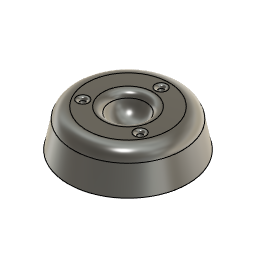
Snap Shine Final Assemply (Autodesk Fusion 360 archive; units mm, degrees)
design "Base"
description: Mounts to wall
Autodesk Fusion 360 part; units mm, degrees
note: some values were not read from the file. Chosen so that the rebuilt part matches the saved one: which bodies a step acts on; a side. Set by a fixed rule: the direction of a hole.
sketch "Sketch3" plane through (0, 0, 0) normal (0, 0, 1) x (1, 0, 0)
  circle A0 centre (0, 0) radius 40
  dimension "d10" = 80
  constraint coincident A0.centre origin
  measures "d10" diameter of A0
ref_plane "WorkPlane2" through (0, 0, 25) normal (0, 0, 1) x (1, 0, 0)
sketch "Sketch5" plane through (0, 0, 25) normal (0, 0, 1) x (1, 0, 0)
  circle A0 centre (0, 0) radius 35
  dimension "d12" = 70
  constraint coincident A0.centre origin
  measures "d12" diameter of A0
loft "Loft1" add profiles "Sketch5", "Sketch3" section 1 section 2
fillet "Fillet4" radius 9 1 edges at (-32.6315, 12.6565, 25)
ref_plane "WorkPlane3" through (0, 0, 25) normal (0, 0, 1) x (1, 0, 0)
sphere "SpherePrimitive2" cut diameter 25 placed x (1, 0, 0) y (0, 1, 0) z (0, 0, 1) at (0, 0, 25)
fillet "Fillet5" radius 5 1 edges at (-4.5202, -11.6541, 25)
sketch "Sketch8" plane through (0, 0, 25) normal (0, 0, 1) x (-1, 0, 0)
  circle A0 centre (0, 0) radius 27.6218
  circle A1 centre (0, 0) radius 16.7705
  circle A2 centre (0, -22.196) radius 1.8885
  circle A3 centre (19.2223, 11.098) radius 1.8885
  circle A4 centre (-19.2223, 11.098) radius 1.8885
  point P0 (19.2223, 11.098)
  point P1 (-19.2223, 11.098)
  dimension "d33" = 3.777
  dimension "d36" = 3.777
  dimension "d37" = 3.777
  dimension "d38" = 22.196
  dimension "d39" = 19.2223
  dimension "d40" = 11.098
  dimension "d41" = 19.2223
  dimension "d42" = 11.098
  constraint coincident P0 A3.centre
  constraint coincident P1 A4.centre
  constraint vertical A0.centre A2.centre
  measures "d33" diameter of A2
  measures "d36" diameter of A3
  measures "d37" diameter of A4
  measures "d38" distance of A0.centre A2.centre
  measures "d39" horizontal distance of A0.centre A3.centre
  measures "d40" vertical distance of A0.centre A3.centre
  measures "d41" horizontal distance of A0.centre P1
  measures "d42" vertical distance of A0.centre P1
extrude "Extrude2" cut sketch "Sketch8" against normal blind 35 contours A2 | A3 | A4
fillet "Fillet6" radius 2 3 edges at (1.7607, 21.5131, 25) (20.983, -11.7809, 25) (-17.4616, -11.7809, 25)
sketch "Sketch11" plane through (0, 0, 0) normal (0, 0, -1) x (1, 0, 0)
  circle A0 centre (0, -22.196) radius 1.8885
  circle A1 centre (19.2223, 11.098) radius 1.8885
  circle A2 centre (-19.2223, 11.098) radius 1.8885
  circle A3 centre (0, 0) radius 40
  line L0 (3.175, 10.175) -> (-3.175, 10.175)
  line L1 (-3.175, 10.175) -> (-3.175, 3.825)
  line L2 (-3.175, 3.825) -> (3.175, 3.825)
  line L3 (3.175, 3.825) -> (3.175, 10.175)
  line L4 (3.175, 10.175) -> (-3.175, 3.825) construction
  line L5 (-3.175, 10.175) -> (3.175, 3.825) construction
  line L6 (-7.2243, -7.8372) -> (-1.725, -4.6622)
  line L7 (-10.3993, -2.3379) -> (-7.2243, -7.8372)
  line L8 (-4.9, 0.8371) -> (-10.3993, -2.3379)
  line L9 (-1.725, -4.6622) -> (-4.9, 0.8371)
  line L10 (10.3993, -2.3378) -> (4.9001, 0.8372)
  line L11 (7.2243, -7.8371) -> (10.3993, -2.3378)
  line L12 (1.7251, -4.6621) -> (7.2243, -7.8371)
  line L13 (4.9001, 0.8372) -> (1.7251, -4.6621)
  point P0 (0, 7)
  point P1 (-6.0622, -3.5)
  point P2 (6.0622, -3.5)
  dimension "d50" = 6.35
  dimension "d51" = 6.35
  dimension "d52" = 7
  dimension "d54" = 360
  constraint horizontal L0
  constraint perpendicular L0 L1
  constraint parallel L0 L2
  constraint parallel L1 L3
  constraint coincident L4 P0
  constraint coincident L5 P0
  measures "d50" distance of L1.end L2.end
  measures "d51" distance of L0.end L1.end
  measures "d52" distance of A3.centre P0
extrude "Extrude4" cut sketch "Sketch11" against normal blind 6.35 contours L0 L1 L2 L3 | L6 L7 L8 L9 | L10 L11 L12 L13

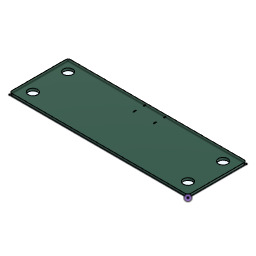
design "circuit board"
description: Cicuit Board for Lamp
Autodesk Fusion 360 part; units mm, degrees
sketch "Sketch1" plane through (0, 0, 0) normal (0, 0, 1) x (1, 0, 0)
  line L0 (0, 0) -> (-76.2, 0)
  line L1 (-76.2, 0) -> (-76.2, 25)
  line L2 (-76.2, 25) -> (0, 25)
  line L3 (0, 25) -> (0, 0)
  dimension "d1" = 76.2
  dimension "d2" = 25
  constraint horizontal L0
  constraint vertical L1
  constraint horizontal L2
  constraint vertical L3
  constraint coincident L0.start L3.end
  measures "d1" distance of L1.end L2.end
  measures "d2" distance of L0.end L1.end
extrude "Extrude1" add sketch "Sketch1" along normal blind 1
fillet "Fillet1" radius 1 4 edges at (0, 0, 0.5) (0, 25, 0.5) (-76.2, 25, 0.5) (-76.2, 0, 0.5)
sketch "Sketch2" plane through (0, 0, 1) normal (0, 0, 1) x (-1, 0, 0)
  arc A0 (76.2, -1) -> (75.2, 0) centre (75.2, -1) ccw
  line L0 (75.2, 0) -> (1, 0)
  arc A1 (1, 0) -> (0, -1) centre (1, -1) ccw
  line L1 (0, -1) -> (0, -24)
  arc A2 (0, -24) -> (1, -25) centre (1, -24) ccw
  line L2 (1, -25) -> (75.2, -25)
  arc A3 (75.2, -25) -> (76.2, -24) centre (75.2, -24) ccw
  line L3 (76.2, -24) -> (76.2, -1)
  point P0 (5, -5)
  dimension "d7" = 5
  dimension "d8" = 5
  measures "d7" horizontal distance of origin P0
  measures "d8" vertical distance of origin P0
hole "Hole1" at (-5, 5, 1) direction (0, 0, -1) diameter 4 end through all
pattern_linear "R-Pattern1" count 2 spacing 66.2 along (-1, 0, 0) count 2 spacing 15 along (0, 1, 0) of "Hole1"
sketch "Sketch5" plane through (0, 0, 0) normal (0, 0, -1) x (1, 0, 0)
  circle A0 centre (-71.2, -20) radius 2
  circle A1 centre (-5, -20) radius 2
  circle A2 centre (-71.2, -5) radius 2
  circle A3 centre (-5, -5) radius 2
  arc A4 (-75.2, 0) -> (-76.2, -1) centre (-75.2, -1) ccw
  line L0 (-76.2, -1) -> (-76.2, -24)
  arc A5 (-76.2, -24) -> (-75.2, -25) centre (-75.2, -24) ccw
  line L1 (-75.2, -25) -> (-1, -25)
  arc A6 (-1, -25) -> (0, -24) centre (-1, -24) ccw
  line L2 (0, -24) -> (0, -1)
  arc A7 (0, -1) -> (-1, 0) centre (-1, -1) ccw
  line L3 (-1, 0) -> (-75.2, 0)
  line L4 (0, -23.5) -> (-76.2, -23.5)
  line L5 (-38.1, -23.5) -> (-42.27, -23.5)
  line L6 (-38.1, -23.5) -> (-33.93, -23.5)
  line L7 (-42.27, -23.5) -> (-42.57, -23.5)
  line L8 (-42.57, -23.5) -> (-42.57, -24.3)
  line L9 (-42.57, -24.3) -> (-42.27, -24.3)
  line L10 (-42.27, -24.3) -> (-42.27, -23.5)
  line L11 (-33.93, -23.5) -> (-33.63, -23.5)
  line L12 (-33.63, -23.5) -> (-33.63, -24.3)
  line L13 (-33.63, -24.3) -> (-33.93, -24.3)
  line L14 (-33.93, -24.3) -> (-33.93, -23.5)
  line L15 (-33.93, -23.5) -> (-33.93, -20.25)
  line L16 (-33.93, -20.25) -> (-33.63, -20.25)
  line L17 (-33.63, -20.25) -> (-33.63, -19.2)
  line L18 (-33.63, -19.2) -> (-33.93, -19.2)
  line L19 (-33.93, -19.2) -> (-33.93, -20.25)
  line L20 (-42.27, -23.5) -> (-42.27, -20.25)
  line L21 (-42.27, -20.25) -> (-42.57, -20.25)
  line L22 (-42.57, -20.25) -> (-42.57, -19.2)
  line L23 (-42.57, -19.2) -> (-42.27, -19.2)
  line L24 (-42.27, -19.2) -> (-42.27, -20.25)
  dimension "d57" = 1.5
  dimension "d58" = 4.17
  dimension "d59" = 4.17
  dimension "d60" = 0.3
  dimension "d61" = 0.8
  dimension "d62" = 0.3
  dimension "d63" = 0.8
  dimension "d64" = 3.25
  dimension "d65" = 0.3
  dimension "d66" = 1.05
  dimension "d67" = 3.25
  dimension "d68" = 0.3
  dimension "d69" = 1.05
  constraint coincident L2 L4.start
  constraint coincident L0 L4.end
  constraint perpendicular L0 L4
  constraint horizontal L5
  constraint midpoint L4 L5.start
  constraint parallel L4 L6
  constraint horizontal L7
  constraint vertical L8
  constraint horizontal L9
  constraint vertical L10
  constraint horizontal L11
  constraint vertical L12
  constraint horizontal L13
  constraint vertical L14
  constraint perpendicular L6 L15
  constraint horizontal L16
  constraint vertical L17
  constraint horizontal L18
  constraint vertical L19
  constraint perpendicular L7 L20
  constraint horizontal L21
  constraint vertical L22
  constraint horizontal L23
  constraint vertical L24
  measures "d57" distance of L1 L4
  measures "d58" distance of L5.start L5.end
  measures "d59" distance of L5.start L6.end
  measures "d60" distance of L5.end L7.end
  measures "d61" distance of L5.end L9.end
  measures "d62" distance of L6.end L11.end
  measures "d63" distance of L6.end L13.end
  measures "d64" distance of L6.end L15.end
  measures "d65" distance of L15.end L16.end
  measures "d66" distance of L15.end L18.end
  measures "d67" distance of L5.end L20.end
  measures "d68" distance of L20.end L21.end
  measures "d69" distance of L20.end L23.end
extrude "Extrude4" cut sketch "Sketch5" against normal through all contours L4 L7 L8 L9 L10 | L4 L11 L12 L13 L14 | L16 L17 L18 L19 | L21 L22 L23 L24

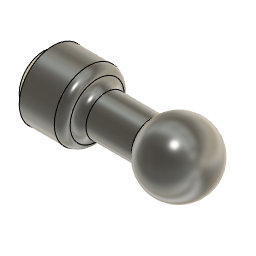
design "Ball Joint"
description: connects to base and lamp
Autodesk Fusion 360 part; units mm, degrees
sketch "Sketch1" plane through (0, 0, 0) normal (1, 0, 0) x (0, 1, 0)
  circle A0 centre (0, 0) radius 12.5
  circle A1 centre (0, 0) radius 9
  dimension "d1" = 25
  dimension "d8" = -3.5
  constraint coincident A0.centre A1.centre
  measures "d1" diameter of A0
extrude "Extrude1" add sketch "Sketch1" along normal blind 20 contours A0 | A1
sketch "Sketch2" plane through (20, 0, 0) normal (1, 0, 0) x (0, 1, 0)
  circle A0 centre (0, 0) radius 12.5
  circle A1 centre (0, 0) radius 7.5
  dimension "d4" = 15
  constraint concentric A0 A1
  measures "d4" diameter of A1
extrude "Extrude2" add sketch "Sketch2" along normal blind 30 contours A1
sphere "SpherePrimitive1" add diameter 25 placed x (0, 1, 0) y (0, 0, 1) z (1, 0, 0) at (50, 0, 0)
extrude "Extrude3" cut sketch "Sketch1" along normal blind 16.5 contours A1
chamfer "Chamfer1" distance 3.5 angle 45 1 edges at (0, -11.6541, -4.5202)
fillet "Fillet1" radius 3.5 1 edges at (20, -11.6541, -4.5202)
fillet "Fillet2" radius 3.5 1 edges at (20, -6.9925, 2.7121)

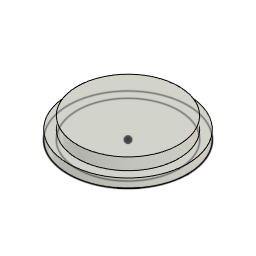
design "LED"
description: light source
Autodesk Fusion 360 part; units mm, degrees
sketch "Sketch1" plane through (0, 0, 0) normal (0, 0, 1) x (1, 0, 0)
  circle A0 centre (0, 0) radius 10
  circle A1 centre (0, 0) radius 8.5
  dimension "d1" = 20
  dimension "d2" = -1.5
  constraint coincident A0.centre A1.centre
  measures "d1" diameter of A0
extrude "Extrude1" add sketch "Sketch1" along normal blind 3.5 contours A1 makes body 1
extrude "Extrude2" add sketch "Sketch1" along normal blind 1.5 bodies 1
sketch "Sketch2" plane through (0, 0, 0) normal (0, 0, 1) x (1, 0, 0)
  line L0 (4.5, -4.5) -> (-4.5, -4.5)
  line L1 (-4.5, -4.5) -> (-4.5, 4.5)
  line L2 (-4.5, 4.5) -> (4.5, 4.5)
  line L3 (4.5, 4.5) -> (4.5, -4.5)
  line L4 (4.5, -4.5) -> (-4.5, 4.5) construction
  line L5 (-4.5, -4.5) -> (4.5, 4.5) construction
  dimension "d7" = 9
  dimension "d8" = 9
  constraint horizontal L0
  constraint perpendicular L0 L1
  constraint parallel L0 L2
  constraint parallel L1 L3
  constraint coincident L4 origin
  constraint coincident L5 origin
  measures "d7" distance of L1.end L2.end
  measures "d8" distance of L0.end L1.end
extrude "Extrude3" add sketch "Sketch2" against normal blind 0.1 separate body makes body 2
equation "d7 = d8"

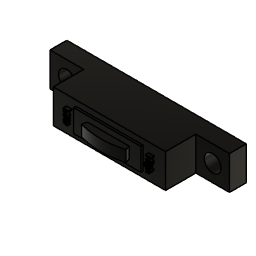
design "Brightness Slider"
description: changes brightness of light
Autodesk Fusion 360 part; units mm, degrees
sketch "Sketch1" plane through (0, 0, 0) normal (0, 1, 0) x (1, 0, 0)
  line L0 (-5, -1.5) -> (5, -1.5)
  line L1 (5, -1.5) -> (5, 1.5)
  line L2 (5, 1.5) -> (-5, 1.5)
  line L3 (-5, 1.5) -> (-5, -1.5)
  line L4 (0, -1.75) -> (0, -22.5)
  line L5 (1.75, 0) -> (22.5, 0)
  line L6 (-3, -1) -> (3, -1)
  line L7 (3, -1) -> (3, 1)
  line L8 (3, 1) -> (-3, 1)
  line L9 (-3, 1) -> (-3, -1)
  line L10 (3.3042, -1) -> (3.3042, 1) construction
  line L11 (3.3042, 1) -> (4, 1) construction
  line L12 (4, 1) -> (4, -1) construction
  line L13 (4, -1) -> (3.3042, -1) construction
  line L14 (-4.0282, -1) -> (-4.0282, 1) construction
  line L15 (-4.0282, 1) -> (-3.3324, 1) construction
  line L16 (-3.3324, 1) -> (-3.3324, -1) construction
  line L17 (-3.3324, -1) -> (-4.0282, -1) construction
  dimension "d1" = 10
  dimension "d2" = 3
  dimension "d3" = 6
  dimension "d4" = 2
  dimension "d5" = 0.5
  dimension "d6" = 0.5
  text T0 "High" font "Arial" height 0.5 align centre top in box 2 x 0.6958 at (3.3042, -1) x (0, 1) y (1, 0) spacing 1
  text T1 "Low\n" font "Arial" height 0.5 align centre top in box 2 x 0.6958 at (-4.0282, -1) x (0, 1) y (1, 0) spacing 1
  constraint horizontal L0
  constraint vertical L1
  constraint horizontal L2
  constraint vertical L3
  constraint symmetric L1 L3 L4
  constraint symmetric L0 L2 L5
  constraint horizontal L6
  constraint vertical L7
  constraint horizontal L8
  constraint vertical L9
  constraint symmetric L4 L7 L9
  constraint symmetric L5 L6 L8
  measures "d1" distance of L1 L3
  measures "d2" distance of L0 L2
  measures "d3" distance of L6.start L6.end
  measures "d4" distance of L6 L8
sketch "Sketch2" plane through (0, 0, 0) normal (0, 1, 0) x (1, 0, 0)
sketch "Sketch3" plane through (0, 0, 0) normal (0, 0, 1) x (1, 0, 0)
extrude "Extrude1" add sketch "Sketch1" against normal blind 0.3 text T1 T0 makes body 1 at (3.9529, -0.1, 0.1717) makes body 2 at (3.7415, -0.2, 0.1717) makes body 3 at (-3.6657, -0.1, 0.6124) makes body 4 at (-3.5909, -0.1, -0.5746) makes body 5 at (-3.6263, 0, 0.229) makes body 6 at (3.7578, -0.1, -0.2788) makes body 7 at (3.6667, -0.1, -0.3716) makes body 8 at (3.6667, -0.1, 0.6666)
extrude "Extrude2" add sketch "Sketch1" along normal blind 2.7 bodies 1 2 3 4 5 6 7 8
extrude "Extrude3" add sketch "Sketch1" against normal blind 0.2 separate body contours L6 L7 L8 L9 makes body 9
sketch "Sketch4" plane through (0, 0, 0) normal (0, 0, 1) x (1, 0, 0)
  arc A0 (-1.8767, -0.6091) -> (2.0803, -0.6091) centre (0.1018, 6.1607) ccw
  constraint horizontal A0.start A0.end
extrude "Extrude4" add sketch "Sketch4" along normal mid plane 1 thin wall 1 on the left open curves A0 bodies 9
sketch "Sketch5" plane through (0, 2.7, 0) normal (0, 1, 0) x (-1, 0, 0)
  line L0 (3, 1) -> (3, -1)
  line L1 (3, -1) -> (-3, -1)
  line L2 (-3, -1) -> (-3, 1)
  line L3 (-3, 1) -> (3, 1)
  line L4 (5, -1.5) -> (5, 1.5)
  line L5 (5, 1.5) -> (-5, 1.5)
  line L6 (-5, 1.5) -> (-5, -1.5)
  line L7 (-5, -1.5) -> (5, -1.5)
  line L8 (-5, 1.5) -> (-8, 1.5)
  line L9 (-8, 1.5) -> (-8, -1.5)
  line L10 (-8, -1.5) -> (-5, -1.5)
  line L11 (-5, -1.5) -> (-5, 1.5)
  line L12 (5, 1.5) -> (8, 1.5)
  line L13 (8, 1.5) -> (8, -1.5)
  line L14 (8, -1.5) -> (5, -1.5)
  line L15 (5, -1.5) -> (5, 1.5)
  line L16 (-8, 1.5) -> (8, 1.5)
  line L17 (8, 1.5) -> (8, -1.5)
  line L18 (8, -1.5) -> (-8, -1.5)
  line L19 (-8, -1.5) -> (-8, 1.5)
  point P0 (-6.5, 0)
  point P1 (6.5, 0)
  dimension "d16" = 3
  dimension "d17" = 3
  dimension "d18" = 3
  dimension "d19" = 1.5
  constraint horizontal L8
  constraint vertical L9
  constraint horizontal L10
  constraint vertical L11
  constraint coincident L5.end L6.start
  constraint horizontal L12
  constraint vertical L13
  constraint horizontal L14
  constraint vertical L15
  constraint coincident L4.end L5.start
  constraint horizontal L16
  constraint vertical L17
  constraint horizontal L18
  constraint vertical L19
  measures "d16" distance of L5.end L8.end
  measures "d17" distance of L4.end L12.end
  measures "d18" distance of L4.end L4.start
  measures "d19" distance of origin L10
extrude "Extrude5" add sketch "Sketch5" along normal blind 1.5 bodies 1
hole "Hole1" at (6.5, 2.7, 0) direction (0, 1, 0) diameter 1.5 depth 2 tip angle 180 bodies 1
hole "Hole2" at (-6.5, 2.7, 0) direction (0, 1, 0) diameter 1.5 depth 2 tip angle 180 bodies 1
scale "Scale1" factor 2 about (3, 0, 1) bodies 1 9

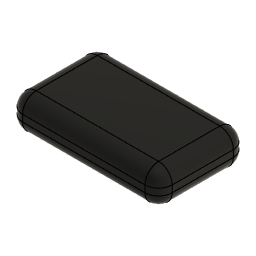
design "Battery"
description: allows lamp to work
Autodesk Fusion 360 part; units mm, degrees
sketch "Sketch1" plane through (0, 0, 0) normal (0, 0, 1) x (1, 0, 0)
  line L0 (22, 13) -> (0, 13)
  line L1 (0, 13) -> (0, 0)
  line L2 (0, 0) -> (22, 0)
  line L3 (22, 0) -> (22, 13)
  dimension "d1" = 22
  dimension "d2" = 13
  constraint horizontal L0
  constraint vertical L1
  constraint horizontal L2
  constraint vertical L3
  constraint coincident L1.end L2.start
  measures "d1" distance of L0.start L0.end
  measures "d2" distance of L0.start L2.end
extrude "Extrude1" add sketch "Sketch1" along normal blind 5
fillet "Fillet1" radius 2 12 edges at (11, 13, 0) (22, 13, 2.5) (0, 13, 2.5) (11, 13, 5) (0, 6.5, 0) (0, 6.5, 5) (11, 0, 0) (11, 0, 5) (22, 6.5, 0) (22, 6.5, 5) (22, 0, 2.5) (0, 0, 2.5)

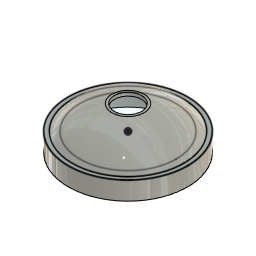
design "Light Reflector"
description: Reflects Light From LED Out
Autodesk Fusion 360 part; units mm, degrees
sketch "Sketch2" plane through (0, 0, 0) normal (1, 0, 0) x (0, 1, 0)
  line L0 (0, 0) -> (34.532, 0)
  arc A0 (34.532, 0) -> (10, 15) centre (-1.0299, -30.5996) ccw
  arc A1 (29.8666, 2) -> (10, 12.9396) centre (-1.0299, -30.5996) ccw
  line L1 (29.8666, 2) -> (29.8666, 0)
  line L2 (10, 15) -> (10, 12.9396)
  line L3 (10, 15) -> (0, 15)
  line L4 (0, 15) -> (0, 0)
  line L5 (10, 12.9396) -> (8.5, 12.9396)
  line L6 (8.5, 12.9396) -> (8.5, 15)
  dimension "d3" = 34.532
  dimension "d6" = 46.9146
  dimension "d29" = 15
  dimension "d30" = 10
  dimension "d32" = 12.9396
  dimension "d33" = 2
  dimension "d34" = 1.5
  constraint coincident L0.start L4.end
  constraint horizontal L0
  constraint concentric A0 A1
  constraint coincident L0 L1.end
  constraint perpendicular L0 L1
  constraint parallel L1 L2
  constraint perpendicular L2 L3
  constraint perpendicular L0 L4
  constraint perpendicular L2 L5
  constraint coincident L3 L6.end
  constraint perpendicular L3 L6
  measures "d3" distance of L0.start L0.end
  measures "d6" radius of A0
  measures "d29" vertical distance of L0.start A0.end
  measures "d30" horizontal distance of L0.start A0.end
  measures "d32" vertical distance of L0.start A1.end
  measures "d33" distance of A1.start L1.end
  measures "d34" distance of A1.end L5.end
revolve "Revolve4" add sketch "Sketch2" angle 360 about axis through (0, 0, 15) along (0, 0, -1) contours L0 A0 A1 L1 L2 | L2 L3 L5 L6
sketch "Sketch5" plane through (0, 0, 0) normal (0, 0, -1) x (1, 0, 0)
  circle A0 centre (0, 0) radius 34.532
  circle A1 centre (0, 0) radius 29.8666
  circle A2 centre (0, 0) radius 34.532
  circle A3 centre (0, 0) radius 37.032
  circle A4 centre (0, 0) radius 29.8666
  dimension "d40" = 2.5
  dimension "d45" = 74.064
  dimension "d46" = 59.7331
  constraint coincident A0.centre A1.centre
  measures "d45" diameter of A3
  measures "d46" diameter of A4
extrude "Extrude3" add sketch "Sketch5" along normal blind 2 contours A0 A2
extrude "Extrude4" add sketch "Sketch5" along normal blind 11.389 contours A3
